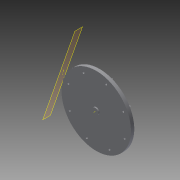
# Autodesk Inventor part: inner bayonet connector 8mk2
Saved by Autodesk Inventor 2015 (Build 190159000, 159)
## iProperties
Created: 2014-09-30
Part Number: inner bayonet connector 8mk2
Material: Generic
Document SubType Name: Modeling
Designer: ericd_000
Density: 1 g/cm^3
Appearance: Default
Author: ericd_000
Autodesk Inventor part; units mm, degrees
ref_plane "YZ Plane" through (0, 0, 0) normal (1, 0, 0) x (0, 1, 0)
ref_plane "XZ Plane" through (0, 0, 0) normal (0, 1, 0) x (-1, 0, 0)
ref_plane "XY Plane" through (0, 0, 0) normal (0, 0, 1) x (1, 0, 0)
sketch "Sketch1" plane through (0, 0, 0) normal (0, 1, 0) x (-1, 0, 0)
  circle A0 centre (0, 0) radius 63
  circle A1 centre (51.0274, 17.6692) radius 2
  circle A2 centre (23.5878, 48.5759) radius 2
  circle A3 centre (-17.6692, 51.0274) radius 2
  circle A4 centre (-48.5759, 23.5878) radius 2
  circle A5 centre (-51.0274, -17.6692) radius 2
  circle A6 centre (-23.5878, -48.5759) radius 2
  circle A7 centre (17.6692, -51.0274) radius 2
  circle A8 centre (48.5759, -23.5878) radius 2
  dimension "d0" = 126
  dimension "d1" = 4
  dimension "d5" = 360
  dimension "d37" = 54
  constraints: 9 centre point, 1 coincident, 17 other
  measures "d0" diameter of A0
  measures "d1" diameter of A1
  measures "d37" distance of A1.centre point (0, 0)
extrude "Extrusion1" add sketch "Sketch1" against normal blind 6
sketch "Sketch4" plane through (0, 0, 0) normal (0, 1, 0) x (1, 0, 0)
  circle A0 centre (-51.0274, -17.6692) radius 2.5
  circle A1 centre (-51.0274, -17.6692) radius 2
  circle A2 centre (-51.0274, -17.6692) radius 2 projected
  point P0 (0, 0)
  dimension "d20" = 5
  dimension "d21" = 4
  constraints: 2 centre point, 2 concentric
  measures "d20" diameter of A0
  measures "d21" diameter of A1
extrude "Extrusion2" add sketch "Sketch4" along normal blind 7.5
sketch "Sketch6" plane through (0, 0, 0) normal (0, 1, 0) x (1, 0, 0)
  line L0 (0, 0) -> (-51.0274, -17.6692) construction
  circle A0 centre (-51.0274, -17.6692) radius 2 construction
  circle A1 centre (-51.0274, -17.6692) radius 3.2389 construction
  line L1 (-51.0274, -17.6692) -> (-63.9956, -22.1597) construction
  line L2 (-64.7566, -29.5758) -> (-68.3351, -19.2414) construction
  constraints: 6 end point, 2 coincident, 1 centre point, 1 collinear, 1 perpendicular
ref_plane "Work Plane1" through (-64.7566, 0, 29.5758) normal (0.9449523, 0, -0.327208) x (-0.327208, 0, -0.9449523)
sketch "Sketch7" plane through (-64.7566, 0, 29.5758) normal (0.9449523, 0, -0.327208) x (-0.327208, 0, -0.9449523)
  line L0 (-56.2411, 0) -> (69.7589, 0) projected
  line L1 (6.7589, 0) -> (6.7589, 6.5)
  line L2 (6.7589, 6.5) -> (12.2106, 6.5)
  line L3 (9.2589, 7.5) -> (4.2589, 7.5) projected
  line L4 (4.2342, 7.5) -> (9.2589, 7.5)
  line L5 (9.2589, 7.5) -> (4.2589, 7.5)
  line L6 (4.2589, 0) -> (4.2589, 7.5) projected
  line L7 (4.2589, 2.9385) -> (9.2589, 7.5)
  constraints: 10 end point, 2 horizontal, 2 point on line
extrude "Extrusion6" cut sketch "Sketch7" along normal blind 20 contours L6 L3 L7 L2 L1 | L1 L2 L7
pattern_circular "Circular Pattern1" count 8 over 360 about axis through (0, 0, 0) along (0, -1, 0) of "Extrusion2", "Extrusion6"
sketch "Sketch5" plane through (0, -6, 0) normal (0, -1, 0) x (1, 0, 0)
  circle A0 centre (0, 0) radius 6
  dimension "d27" = 12
  constraints: 1 centre point, 1 coincident
  measures "d27" diameter of A0
extrude "Extrusion3" add sketch "Sketch5" along normal blind 2
ref_plane "Work Plane2" through (-66.7031, 0, -24.8766) normal (0.8995532, 0, 0.4368112) x (0.4368112, 0, -0.8995532)
ref_plane "Work Plane3" through (-29.5758, 0, -64.7566) normal (0.327208, 0, 0.9449523) x (0.9449523, 0, -0.327208)
ref_plane "Work Plane4" through (24.8766, 0, -66.7031) normal (-0.4368112, 0, 0.8995532) x (0.8995532, 0, 0.4368112)
ref_plane "Work Plane5" through (64.7566, 0, -29.5758) normal (-0.9449523, 0, 0.327208) x (0.327208, 0, 0.9449523)
ref_plane "Work Plane6" through (66.7031, 0, 24.8766) normal (-0.8995532, 0, -0.4368112) x (-0.4368112, 0, 0.8995532)
ref_plane "Work Plane7" through (29.5758, 0, 64.7566) normal (-0.327208, 0, -0.9449523) x (-0.9449523, 0, 0.327208)
ref_plane "Work Plane8" through (-24.8766, 0, 66.7031) normal (0.4368112, 0, -0.8995532) x (-0.8995532, 0, -0.4368112)
body "Solid1"
